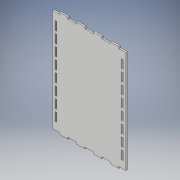
# Autodesk Inventor part: 1 binnen achterplaat
Saved by Autodesk Inventor 2019 (Build 230136000, 136)
## iProperties
Created: 2021-01-09
Part Number: 1 binnen achterplaat
Material: Generic
Document SubType Name: Sheet Metal
Designer: Stefan
Density: 1 g/cm^3
Sheet Metal Rule: Default_mm
Appearance: Default
Author: Stefan
Autodesk Inventor part; units mm, degrees
ref_plane "YZ Plane" through (0, 0, 0) normal (1, 0, 0) x (0, 1, 0)
ref_plane "XZ Plane" through (0, 0, 0) normal (0, 1, 0) x (-1, 0, 0)
ref_plane "XY Plane" through (0, 0, 0) normal (0, 0, 1) x (1, 0, 0)
sketch "Sketch1" plane through (0, 0, 0) normal (0, 0, 1) x (1, 0, 0)
  line L0 (-65, -90.5) -> (65, -90.5)
  line L1 (65, -90.5) -> (65, 90.5)
  line L2 (65, 90.5) -> (-65, 90.5)
  line L3 (-65, 90.5) -> (-65, -90.5)
  line L4 (-65, -90.5) -> (65, 90.5) construction
  line L5 (65, -90.5) -> (-65, 90.5) construction
  line L6 (-60, 77.5) -> (-57, 77.5)
  line L7 (-57, 77.5) -> (-57, 62.5)
  line L8 (-57, 62.5) -> (-60, 62.5)
  line L9 (-60, 62.5) -> (-60, 77.5)
  line L10 (-60, 77.5) -> (-57, 62.5) construction
  line L11 (-57, 77.5) -> (-60, 62.5) construction
  line L12 (-60, 57.5) -> (-57, 57.5)
  line L13 (-57, 57.5) -> (-57, 42.5)
  line L14 (-57, 42.5) -> (-60, 42.5)
  line L15 (-60, 42.5) -> (-60, 57.5)
  line L16 (-60, 57.5) -> (-57, 42.5) construction
  line L17 (-57, 57.5) -> (-60, 42.5) construction
  line L18 (-60, 37.5) -> (-57, 37.5)
  line L19 (-57, 37.5) -> (-57, 22.5)
  line L20 (-57, 22.5) -> (-60, 22.5)
  line L21 (-60, 22.5) -> (-60, 37.5)
  line L22 (-60, 37.5) -> (-57, 22.5) construction
  line L23 (-57, 37.5) -> (-60, 22.5) construction
  line L24 (-60, 17.5) -> (-57, 17.5)
  line L25 (-57, 17.5) -> (-57, 2.5)
  line L26 (-57, 2.5) -> (-60, 2.5)
  line L27 (-60, 2.5) -> (-60, 17.5)
  line L28 (-60, 17.5) -> (-57, 2.5) construction
  line L29 (-57, 17.5) -> (-60, 2.5) construction
  line L30 (-60, -2.5) -> (-57, -2.5)
  line L31 (-57, -2.5) -> (-57, -17.5)
  line L32 (-57, -17.5) -> (-60, -17.5)
  line L33 (-60, -17.5) -> (-60, -2.5)
  line L34 (-60, -2.5) -> (-57, -17.5) construction
  line L35 (-57, -2.5) -> (-60, -17.5) construction
  line L36 (-60, -22.5) -> (-57, -22.5)
  line L37 (-57, -22.5) -> (-57, -37.5)
  line L38 (-57, -37.5) -> (-60, -37.5)
  line L39 (-60, -37.5) -> (-60, -22.5)
  line L40 (-60, -22.5) -> (-57, -37.5) construction
  line L41 (-57, -22.5) -> (-60, -37.5) construction
  line L42 (-60, -42.5) -> (-57, -42.5)
  line L43 (-57, -42.5) -> (-57, -57.5)
  line L44 (-57, -57.5) -> (-60, -57.5)
  line L45 (-60, -57.5) -> (-60, -42.5)
  line L46 (-60, -42.5) -> (-57, -57.5) construction
  line L47 (-57, -42.5) -> (-60, -57.5) construction
  line L48 (-60, -62.5) -> (-57, -62.5)
  line L49 (-57, -62.5) -> (-57, -77.5)
  line L50 (-57, -77.5) -> (-60, -77.5)
  line L51 (-60, -77.5) -> (-60, -62.5)
  line L52 (-60, -62.5) -> (-57, -77.5) construction
  line L53 (-57, -62.5) -> (-60, -77.5) construction
  line L54 (57, 77.5) -> (60, 77.5)
  line L55 (60, 77.5) -> (60, 62.5)
  line L56 (60, 62.5) -> (57, 62.5)
  line L57 (57, 62.5) -> (57, 77.5)
  line L58 (57, 77.5) -> (60, 62.5) construction
  line L59 (60, 77.5) -> (57, 62.5) construction
  line L60 (57, 57.5) -> (60, 57.5)
  line L61 (60, 57.5) -> (60, 42.5)
  line L62 (60, 42.5) -> (57, 42.5)
  line L63 (57, 42.5) -> (57, 57.5)
  line L64 (57, 57.5) -> (60, 42.5) construction
  line L65 (60, 57.5) -> (57, 42.5) construction
  line L66 (57, 37.5) -> (60, 37.5)
  line L67 (60, 37.5) -> (60, 22.5)
  line L68 (60, 22.5) -> (57, 22.5)
  line L69 (57, 22.5) -> (57, 37.5)
  line L70 (57, 37.5) -> (60, 22.5) construction
  line L71 (60, 37.5) -> (57, 22.5) construction
  line L72 (57, 17.5) -> (60, 17.5)
  line L73 (60, 17.5) -> (60, 2.5)
  line L74 (60, 2.5) -> (57, 2.5)
  line L75 (57, 2.5) -> (57, 17.5)
  line L76 (57, 17.5) -> (60, 2.5) construction
  line L77 (60, 17.5) -> (57, 2.5) construction
  line L78 (57, -2.5) -> (60, -2.5)
  line L79 (60, -2.5) -> (60, -17.5)
  line L80 (60, -17.5) -> (57, -17.5)
  line L81 (57, -17.5) -> (57, -2.5)
  line L82 (57, -2.5) -> (60, -17.5) construction
  line L83 (60, -2.5) -> (57, -17.5) construction
  line L84 (57, -22.5) -> (60, -22.5)
  line L85 (60, -22.5) -> (60, -37.5)
  line L86 (60, -37.5) -> (57, -37.5)
  line L87 (57, -37.5) -> (57, -22.5)
  line L88 (57, -22.5) -> (60, -37.5) construction
  line L89 (60, -22.5) -> (57, -37.5) construction
  line L90 (57, -42.5) -> (60, -42.5)
  line L91 (60, -42.5) -> (60, -57.5)
  line L92 (60, -57.5) -> (57, -57.5)
  line L93 (57, -57.5) -> (57, -42.5)
  line L94 (57, -42.5) -> (60, -57.5) construction
  line L95 (60, -42.5) -> (57, -57.5) construction
  line L96 (57, -62.5) -> (60, -62.5)
  line L97 (60, -62.5) -> (60, -77.5)
  line L98 (60, -77.5) -> (57, -77.5)
  line L99 (57, -77.5) -> (57, -62.5)
  line L100 (57, -62.5) -> (60, -77.5) construction
  line L101 (60, -62.5) -> (57, -77.5) construction
  point P0 (0, 0)
  point P1 (-58.5, 70)
  point P2 (-58.5, 50)
  point P3 (-58.5, 30)
  point P4 (-58.5, 10)
  point P5 (-58.5, -10)
  point P6 (-58.5, -30)
  point P7 (-58.5, -50)
  point P8 (-58.5, -70)
  point P9 (58.5, 70)
  point P10 (58.5, 50)
  point P11 (58.5, 30)
  point P12 (58.5, 10)
  point P13 (58.5, -10)
  point P14 (58.5, -30)
  point P15 (58.5, -50)
  point P16 (58.5, -70)
  dimension "d0" = 130
  dimension "d1" = 181
  dimension "d2" = 3
  dimension "d3" = 15
  dimension "d8" = 5
  dimension "d9" = 13
  dimension "d12" = 20
  dimension "d15" = 117
  constraints: 204 end point, 34 midpoint, 4 parallel, 3 horizontal, 2 perpendicular, 1 vertical, 165 other
  measures "d0" distance of L2.end L1.end
  measures "d1" distance of L0.end L1.end
  measures "d2" distance of L7.end L8.end
  measures "d3" distance of L6.end L7.end
  measures "d8" distance between parallel lines of L3 L9
  measures "d9" distance between parallel lines of L2 L6
  measures "d12" distance of L6.start L12.start
  measures "d15" distance of L6.start L54.start
extrude "Extrusion1" add sketch "Sketch1" along normal blind 3
sketch "Sketch2" plane through (0, 0, 3) normal (0, 0, 1) x (1, 0, 0)
  line L0 (65, 90.5) -> (-65, 90.5) projected
  line L1 (-52.5, 90.5) -> (-37.5, 90.5)
  line L2 (-37.5, 90.5) -> (-37.5, 93.5)
  line L3 (-37.5, 93.5) -> (-52.5, 93.5)
  line L4 (-52.5, 93.5) -> (-52.5, 90.5)
  line L5 (-22.5, 90.5) -> (-7.5, 90.5)
  line L6 (-7.5, 90.5) -> (-7.5, 93.5)
  line L7 (-7.5, 93.5) -> (-22.5, 93.5)
  line L8 (-22.5, 93.5) -> (-22.5, 90.5)
  line L9 (7.5, 90.5) -> (22.5, 90.5)
  line L10 (22.5, 90.5) -> (22.5, 93.5)
  line L11 (22.5, 93.5) -> (7.5, 93.5)
  line L12 (7.5, 93.5) -> (7.5, 90.5)
  line L13 (37.5, 90.5) -> (52.5, 90.5)
  line L14 (52.5, 90.5) -> (52.5, 93.5)
  line L15 (52.5, 93.5) -> (37.5, 93.5)
  line L16 (37.5, 93.5) -> (37.5, 90.5)
  line L17 (-52.5, -93.5) -> (-37.5, -93.5)
  line L18 (-37.5, -93.5) -> (-37.5, -90.5)
  line L19 (-37.5, -90.5) -> (-52.5, -90.5)
  line L20 (-52.5, -90.5) -> (-52.5, -93.5)
  line L21 (-22.5, -93.5) -> (-7.5, -93.5)
  line L22 (-7.5, -93.5) -> (-7.5, -90.5)
  line L23 (-7.5, -90.5) -> (-22.5, -90.5)
  line L24 (-22.5, -90.5) -> (-22.5, -93.5)
  line L25 (7.5, -93.5) -> (22.5, -93.5)
  line L26 (22.5, -93.5) -> (22.5, -90.5)
  line L27 (22.5, -90.5) -> (7.5, -90.5)
  line L28 (7.5, -90.5) -> (7.5, -93.5)
  line L29 (37.5, -93.5) -> (52.5, -93.5)
  line L30 (52.5, -93.5) -> (52.5, -90.5)
  line L31 (52.5, -90.5) -> (37.5, -90.5)
  line L32 (37.5, -90.5) -> (37.5, -93.5)
  line L33 (-65, 90.5) -> (-65, -90.5) projected
  point P0 (0, 0)
  dimension "d20" = 15
  dimension "d21" = 3
  dimension "d24" = 30
  dimension "d27" = 184
  dimension "d30" = 12.5
  constraints: 64 end point, 2 collinear, 2 horizontal, 2 parallel, 1 perpendicular, 1 point on line, 1 vertical, 54 other
  measures "d20" distance of L3.end L2.end
  measures "d21" distance of L2.end L1.end
  measures "d24" distance of L1.start L5.start
  measures "d27" distance of L1.start L17.start
  measures "d30" distance between parallel lines of L33 L4
extrude "Extrusion2" add sketch "Sketch2" against normal blind 3
equation "\"BendRadius\" = Thickness"
equation "\"BendReliefWidth\" = Thickness"
equation "\"BendReliefDepth\" = 0.5 * Thickness"
equation "\"CornerReliefSize\" = 4 * Thickness"
equation "\"MinimumRemnant\" = 2 * Thickness"
equation "\"TransitionRadius\" = BendRadius"
equation "\"JacobiRadiusSize\" = BendRadius"
equation "\"GapSize\" = Thickness"
equation "\"Thickness\" = 0.5"
body "Solid1"
